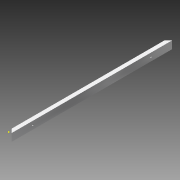
# Autodesk Inventor part: 42in 2x1 boxbeam
Saved by Autodesk Inventor 2015 (Build 190159000, 159)
## iProperties
Created: 2015-01-11
Part Number: 42in 2x1 boxbeam
Material: Generic
Document SubType Name: Modeling
Designer: chapale16
Density: 1 g/cm^3
Appearance: Chrome - Polished
Author: chapale16
Autodesk Inventor part; units mm, degrees
ref_plane "YZ Plane" through (0, 0, 0) normal (1, 0, 0) x (0, 1, 0)
ref_plane "XZ Plane" through (0, 0, 0) normal (0, 1, 0) x (-1, 0, 0)
ref_plane "XY Plane" through (0, 0, 0) normal (0, 0, 1) x (1, 0, 0)
sketch "Sketch2" plane through (0, 0, 0) normal (0, 0, 1) x (1, 0, 0)
  line L0 (-4.1078, 5.9023) -> (21.2922, 5.9023)
  line L1 (21.2922, 5.9023) -> (21.2922, -44.8977)
  line L2 (21.2922, -44.8977) -> (-4.1078, -44.8977)
  line L3 (-4.1078, -44.8977) -> (-4.1078, 5.9023)
  line L4 (18.1934, 2.8035) -> (-1.009, 2.8035)
  line L5 (-1.009, 2.8035) -> (-1.009, -41.7989)
  line L6 (-1.009, -41.7989) -> (18.1934, -41.7989)
  line L7 (18.1934, -41.7989) -> (18.1934, 2.8035)
  point P0 (0, 0)
  dimension "d0" = 25.4
  dimension "d1" = 50.8
  dimension "d2" = 3.0988
  constraints: 16 end point, 4 parallel, 2 perpendicular, 1 horizontal, 3 other
  measures "d0" distance of L1.end L2.end
  measures "d1" distance of L0.end L1.end
  measures "d2" distance between parallel lines of L0 L4
extrude "Extrusion1" add sketch "Sketch2" along normal blind 1066.8
sketch "Sketch5" plane through (0, 0, 1066.8) normal (0, 0, 1) x (1, 0, 0)
  point P0 (0, 0)
sketch "Sketch6" plane through (-4.1078, 5.9023, 0) normal (0, 1, 0) x (1, 0, 0)
  line L0 (25.4, 0) -> (-1.2066, -26.6066)
  line L1 (0, 0) -> (0, -1066.8) projected
  line L2 (0, -25.4) -> (0, 0)
  line L3 (0, 0) -> (25.4, 0)
  line L4 (0, -1066.8) -> (25.4, -1066.8) projected
  line L5 (25.4, -1066.8) -> (-7.0638, -1034.3362)
  line L6 (25.4, -1066.8) -> (71.3108, -1066.8) construction
  line L7 (0, -1041.4) -> (0, -1066.8)
  line L8 (0, -1066.8) -> (25.4, -1066.8)
  point P0 (4.1078, 0)
  dimension "d11" = 135
  constraints: 14 end point, 4 point on line, 2 perpendicular, 1 collinear, 1 equal length, 1 horizontal, 1 vertical
  measures "d11" angle of L6 L5
extrude "Extrusion2" cut sketch "Sketch6" against normal blind 1066.8 contours L0 L1 L3
extrude "Extrusion3" cut sketch "Sketch6" against normal blind 1066.8 contours L5 L4 L1
sketch "Sketch7" plane through (21.2922, -44.8977, 0) normal (1, 0, 0) x (0, 0, -1)
  line L0 (0, 0) -> (-1066.8, 0) projected
  line L1 (0, 50.4825) -> (-139.7, 50.4825)
  line L2 (-139.7, 50.4825) -> (-139.7, 0)
  line L3 (-139.7, 0) -> (0, 0)
  line L4 (0, 0) -> (0, 50.4825)
  line L5 (-1066.8, 50.4825) -> (-927.1, 50.4825)
  line L6 (-927.1, 50.4825) -> (-927.1, -0.3175)
  line L7 (-927.1, -0.3175) -> (-1066.8, -0.3175)
  line L8 (-1066.8, -0.3175) -> (-1066.8, 50.4825)
  point P0 (0, 44.8977)
  point P1 (-139.7, 25.2412)
  point P2 (-927.1, 25.0825)
  dimension "d12" = 139.7
  dimension "d13" = 139.7
  dimension "d14" = 50.8
  constraints: 16 end point, 4 parallel, 2 horizontal, 2 midpoint, 2 perpendicular, 1 point on line
  measures "d12" distance of L3.end L2.end
  measures "d13" distance of L6.end L7.end
  measures "d14" distance of L5.end L6.end
hole "Hole1" at (21.2922, -19.8152, 927.1) at (21.2922, -19.6564, 139.7) direction (-1, 0, 0) diameter 9.525 end through all
body "Solid1"
